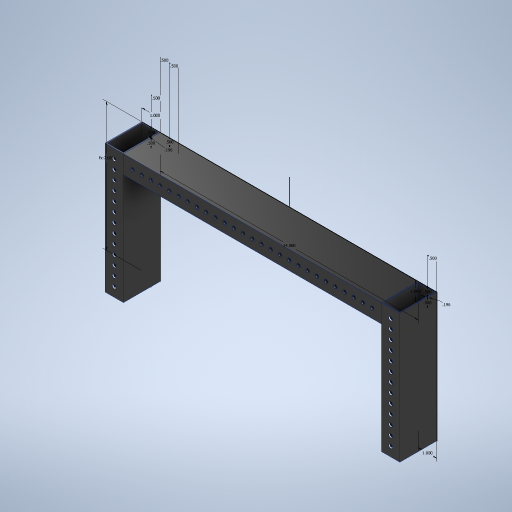
# Autodesk Inventor part: 2024-220-000-Hard-Stop
Saved by Autodesk Inventor 2024 (Build 280153000, 153)
## iProperties
Created: 2024-01-23
Part Number: 2024-220-000-Hard-Stop
Material: Aluminum 6061
Document SubType Name: Modeling
Designer: rohan
Density: 2.7 g/cm^3
Appearance: Aluminum - Flat
Author: rohan
Autodesk Inventor part; units mm, degrees
ref_plane "YZ Plane" through (0, 0, 0) normal (1, 0, 0) x (0, 1, 0)
ref_plane "XZ Plane" through (0, 0, 0) normal (0, 1, 0) x (-1, 0, 0)
ref_plane "XY Plane" through (0, 0, 0) normal (0, 0, 1) x (1, 0, 0)
sketch "Sketch1" plane through (0, 0, 0) normal (0, 0, 1) x (1, 0, 0)
  line L0 (0, 0) -> (25.4, 0)
  line L1 (25.4, 0) -> (25.4, 177.8)
  line L2 (25.4, 177.8) -> (0, 177.8)
  line L3 (0, 177.8) -> (0, 0)
  line L4 (25.4, 177.8) -> (381, 177.8)
  line L5 (381, 177.8) -> (381, 152.4)
  line L6 (381, 152.4) -> (25.4, 152.4)
  line L7 (25.4, 152.4) -> (25.4, 177.8)
  line L8 (381, 177.8) -> (406.4, 177.8)
  line L9 (406.4, 177.8) -> (406.4, 0)
  line L10 (406.4, 0) -> (381, 0)
  line L11 (381, 0) -> (381, 177.8)
  circle A0 centre (38.1, 165.1) radius 2.4892
  circle A1 centre (50.8, 165.1) radius 2.4892
  circle A2 centre (63.5, 165.1) radius 2.4892
  circle A3 centre (76.2, 165.1) radius 2.4892
  circle A4 centre (88.9, 165.1) radius 2.4892
  circle A5 centre (101.6, 165.1) radius 2.4892
  circle A6 centre (114.3, 165.1) radius 2.4892
  circle A7 centre (127, 165.1) radius 2.4892
  circle A8 centre (139.7, 165.1) radius 2.4892
  circle A9 centre (152.4, 165.1) radius 2.4892
  circle A10 centre (165.1, 165.1) radius 2.4892
  circle A11 centre (177.8, 165.1) radius 2.4892
  circle A12 centre (190.5, 165.1) radius 2.4892
  circle A13 centre (203.2, 165.1) radius 2.4892
  circle A14 centre (215.9, 165.1) radius 2.4892
  circle A15 centre (228.6, 165.1) radius 2.4892
  circle A16 centre (241.3, 165.1) radius 2.4892
  circle A17 centre (254, 165.1) radius 2.4892
  circle A18 centre (266.7, 165.1) radius 2.4892
  circle A19 centre (279.4, 165.1) radius 2.4892
  circle A20 centre (292.1, 165.1) radius 2.4892
  circle A21 centre (304.8, 165.1) radius 2.4892
  circle A22 centre (317.5, 165.1) radius 2.4892
  circle A23 centre (330.2, 165.1) radius 2.4892
  circle A24 centre (342.9, 165.1) radius 2.4892
  circle A25 centre (355.6, 165.1) radius 2.4892
  circle A26 centre (368.3, 165.1) radius 2.4892
  line L12 (203.2, 177.8) -> (203.2, 213.6328)
  circle A27 centre (12.7, 165.1) radius 2.4892
  circle A28 centre (12.7, 152.4) radius 2.4892
  circle A29 centre (12.7, 139.7) radius 2.4892
  circle A30 centre (12.7, 127) radius 2.4892
  circle A31 centre (12.7, 114.3) radius 2.4892
  circle A32 centre (12.7, 101.6) radius 2.4892
  circle A33 centre (12.7, 88.9) radius 2.4892
  circle A34 centre (12.7, 76.2) radius 2.4892
  circle A35 centre (12.7, 63.5) radius 2.4892
  circle A36 centre (393.7, 165.1) radius 2.4892
  circle A37 centre (393.7, 152.4) radius 2.4892
  circle A38 centre (393.7, 139.7) radius 2.4892
  circle A39 centre (393.7, 127) radius 2.4892
  circle A40 centre (393.7, 114.3) radius 2.4892
  circle A41 centre (393.7, 101.6) radius 2.4892
  circle A42 centre (393.7, 88.9) radius 2.4892
  circle A43 centre (393.7, 76.2) radius 2.4892
  circle A44 centre (393.7, 63.5) radius 2.4892
  circle A45 centre (393.7, 50.8) radius 2.4892
  circle A46 centre (393.7, 38.1) radius 2.4892
  circle A47 centre (393.7, 25.4) radius 2.4892
  circle A48 centre (393.7, 12.7) radius 2.4892
  circle A49 centre (12.7, 50.8) radius 2.4892
  circle A50 centre (12.7, 38.1) radius 2.4892
  circle A51 centre (12.7, 25.4) radius 2.4892
  circle A52 centre (12.7, 12.7) radius 2.4892
  point P0 (25.4, 165.1)
  point P1 (12.7, -12.7)
  point P2 (25.4, 152.4)
  point P3 (12.7, 177.8)
  point P4 (393.7, 177.8)
  dimension "d0" = 25.4
  dimension "d2" = 355.6
  dimension "d3" = 25.4
  dimension "d4" = 25.4
  dimension "d64" = 12.7
  dimension "d65" = 12.7
  dimension "d68" = 12.7
  dimension "d73" = 177.8
  dimension "d75" = 4.9784
  dimension "d76" = 12.7
  dimension "d77" = 12.7
  dimension "d80" = 12.7
  dimension "d85" = 4.9784
  dimension "d86" = 12.7
  dimension "d87" = 12.7
  dimension "d90" = 12.7
  constraints: 53 centre point, 26 end point, 6 parallel, 4 horizontal, 4 midpoint, 3 perpendicular, 3 vertical, 1 point on line, 100 other
  measures "d0" distance of L2.end L1.end
  measures "d2" distance of L5.end L6.end
  measures "d3" distance of L4.end L5.end
  measures "d4" distance of L9.end L10.end
  measures "d64" distance from line of L7 A0.centre
  measures "d65" distance from line of L4 A0.centre
  measures "d68" distance of A0.centre A1.centre
  measures "d73" distance of L2.end L0.start
  measures "d75" diameter of A27
  measures "d76" distance from line of A27.centre L1
  measures "d77" distance of point (12.7, 177.8) A27.centre
  measures "d80" distance of A27.centre A28.centre
  measures "d85" diameter of A36
  measures "d86" distance of point (393.7, 177.8) A36.centre
  measures "d87" distance from line of L9 A36.centre
  measures "d90" distance of A36.centre A37.centre
extrude "Extrusion1" add sketch "Sketch1" along normal blind 50.8 contours L3 L2 L1 L0 | A27 | A28 | A29 | A30 | A31 | A32 | A33 | A34 | A35 | A49 | A50 | A51 | A52
extrude "Extrusion2" add sketch "Sketch1" along normal blind 50.8 separate body contours L1 L4 L5 L6
extrude "Extrusion3" add sketch "Sketch1" along normal blind 50.8 separate body contours L5 L8 L9 L10 L11 | A36 | A37 | A38 | A39 | A40 | A41 | A42 | A43 | A44 | A45 | A46 | A47 | A48
sketch "Sketch2" plane through (0, 177.8, 0) normal (0, 1, 0) x (1, 0, 0)
  line L0 (25.4, 0) -> (0, 0) projected
  line L1 (0, 0) -> (0, -50.8) projected
  line L2 (25.4, -50.8) -> (0, -50.8) projected
  line L3 (25.4, 0) -> (25.4, -50.8) projected
  line L4 (23.8125, -49.2125) -> (1.5875, -49.2125)
  line L5 (1.5875, -49.2125) -> (1.5875, -1.5875)
  line L6 (1.5875, -1.5875) -> (23.8125, -1.5875)
  line L7 (23.8125, -1.5875) -> (23.8125, -49.2125)
  point P0 (0, 0)
  dimension "d38" = 1.5875
  constraints: 8 end point, 3 other
  measures "d38" distance between parallel lines of L3 L7
extrude "Extrusion4" cut sketch "Sketch2" against normal blind 322.2625 contours L4 L5 L6 L7 bodies 1
sketch "Sketch3" plane through (381, 177.8, 0) normal (0, 1, 0) x (1, 0, 0)
  line L0 (25.4, 0) -> (0, 0) projected
  line L1 (0, 0) -> (0, -50.8) projected
  line L2 (25.4, -50.8) -> (0, -50.8) projected
  line L3 (25.4, 0) -> (25.4, -50.8) projected
  line L4 (23.8125, -49.2125) -> (1.5875, -49.2125)
  line L5 (1.5875, -49.2125) -> (1.5875, -1.5875)
  line L6 (1.5875, -1.5875) -> (23.8125, -1.5875)
  line L7 (23.8125, -1.5875) -> (23.8125, -49.2125)
  point P0 (-381, 0)
  dimension "d41" = 1.5875
  constraints: 8 end point, 3 other
  measures "d41" distance between parallel lines of L3 L7
extrude "Extrusion5" cut sketch "Sketch3" against normal blind 322.2625 contours L4 L5 L6 L7 bodies 3
sketch "Sketch4" plane through (381, 152.4, 0) normal (1, 0, 0) x (0, 0, -1)
  line L0 (0, 0) -> (0, 25.4) projected
  line L1 (0, 25.4) -> (-50.8, 25.4) projected
  line L2 (-50.8, 0) -> (-50.8, 25.4) projected
  line L3 (0, 0) -> (-50.8, 0) projected
  line L4 (-49.2125, 23.8125) -> (-1.5875, 23.8125)
  line L5 (-1.5875, 23.8125) -> (-1.5875, 1.5875)
  line L6 (-1.5875, 1.5875) -> (-49.2125, 1.5875)
  line L7 (-49.2125, 1.5875) -> (-49.2125, 23.8125)
  point P0 (0, -152.4)
  dimension "d44" = 1.5875
  constraints: 8 end point, 3 other
  measures "d44" distance between parallel lines of L2 L7
extrude "Extrusion6" cut sketch "Sketch4" against normal blind 279.4 contours L4 L5 L6 L7 bodies 2
sketch "Sketch5" plane through (25.4, 152.4, 0) normal (-1, 0, 0) x (0, 0, 1)
  line L0 (0, 25.4) -> (0, 0) projected
  line L1 (0, 0) -> (50.8, 0) projected
  line L2 (50.8, 25.4) -> (50.8, 0) projected
  line L3 (0, 25.4) -> (50.8, 25.4) projected
  line L4 (49.2125, 23.8125) -> (49.2125, 1.5875)
  line L5 (49.2125, 1.5875) -> (1.5875, 1.5875)
  line L6 (1.5875, 1.5875) -> (1.5875, 23.8125)
  line L7 (1.5875, 23.8125) -> (49.2125, 23.8125)
  point P0 (0, -152.4)
  dimension "d54" = 1.5875
  constraints: 8 end point, 3 other
  measures "d54" distance between parallel lines of L3 L7
extrude "Extrusion7" cut sketch "Sketch5" against normal blind 119.0625 contours L4 L5 L6 L7 bodies 2
extrude "Extrusion8" cut sketch "Sketch1" along normal blind 63.5 contours A36 | A37 | A38 | A39 | A40 | A41 | A42 | A43 | A44 | A45 | A46 | A47 | A48 bodies 3
extrude "Extrusion9" cut sketch "Sketch1" along normal blind 63.5 contours A27 | A28 | A29 | A30 | A31 | A32 | A33 | A34 | A35 | A49 | A50 | A51 | A52 bodies 1
equation "\"d73\" = Height"
equation "\"Height\" = 177.8"
